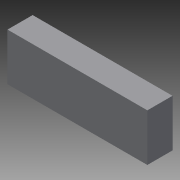
# Autodesk Inventor part: lipo2s
Saved by Autodesk Inventor 2015 (Build 190159000, 159)
## iProperties
Created: 2015-08-03
Part Number: lipo2s
Material: Générique
Document SubType Name: Modeling
Designer: astralien3000
Density: 1 g/cm^3
Appearance: Par défaut
Author: astralien3000
Autodesk Inventor part; units mm, degrees
ref_plane "YZ Plane" through (0, 0, 0) normal (1, 0, 0) x (0, 1, 0)
ref_plane "XZ Plane" through (0, 0, 0) normal (0, 1, 0) x (-1, 0, 0)
ref_plane "XY Plane" through (0, 0, 0) normal (0, 0, 1) x (1, 0, 0)
sketch "Esquisse1" plane through (0, 0, 0) normal (0, 1, 0) x (-1, 0, 0)
  line L0 (-69.5, 23.5) -> (69.5, 23.5)
  line L1 (69.5, 23.5) -> (69.5, -23.5)
  line L2 (69.5, -23.5) -> (-69.5, -23.5)
  line L3 (-69.5, -23.5) -> (-69.5, 23.5)
  point P0 (0, 0)
  dimension "d0" = 139
  dimension "d1" = 47
  dimension "d2" = 23.5
  dimension "d3" = 69.5
  constraints: 8 end point, 2 parallel, 1 horizontal, 1 perpendicular
  measures "d0" distance of L0.start L0.end
  measures "d1" distance of L2.end L0.start
  measures "d2" distance from line of L0 point (0, 0)
  measures "d3" distance from line of point (0, 0) L1
extrude "Extrusion1" add sketch "Esquisse1" along normal blind 25
equation "\"d2\" = 0.5 * d1"
equation "\"d3\" = 0.5 * d0"
